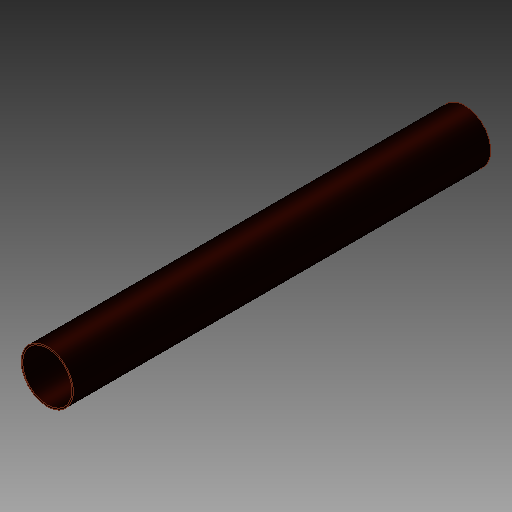
# Autodesk Inventor part: 2210_Copper Bore_V1
Saved by Autodesk Inventor 2020 (Build 240168000, 168)
## iProperties
Created: 2017-06-05
Part Number: 2210_Copper Bore_V1
Material: Copper
Document SubType Name: Modeling
Designer: MPI
Density: 8.94 g/cm^3
Appearance: Copper - Satin
Mass: 9061.06 g
Surface Area: 6406.68 cm^2
Volume: 1013.54 cm^3
Author: MPI
Autodesk Inventor part; units mm, degrees
ref_plane "YZ Plane" through (0, 0, 0) normal (1, 0, 0) x (0, 1, 0)
ref_plane "XZ Plane" through (0, 0, 0) normal (0, 1, 0) x (-1, 0, 0)
ref_plane "XY Plane" through (0, 0, 0) normal (0, 0, 1) x (1, 0, 0)
sketch "Sketch1" plane through (0, 0, 0) normal (0, 1, 0) x (-1, 0, 0)
  circle A0 centre (0, 0) radius 57.15
  circle A1 centre (0, 0) radius 53.975
  dimension "d0" = 114.3
  dimension "d1" = 107.95
  constraints: 2 centre point, 2 coincident
  measures "d0" diameter of A0
  measures "d1" diameter of A1
extrude "Extrusion1" add sketch "Sketch1" along normal mid plane 914.4
body "Solid1"
